Autodesk Inventor part; units mm, degrees
(part 5 of 13)
  line L1929 (20.935, 0.83) -> (20.6882, 0.83) construction
  spline S605 degree 3 poles (20.6882, 0.83) (20.4415, 0.83) (20.2414, 0.6299) (20.2414, 0.3832) knots 0 0 0 0 1 1 1 1
  line L1930 (20.6882, 0.83) -> (20.4415, 0.83) construction
  line L1931 (20.4415, 0.83) -> (20.2414, 0.6299) construction
  line L1932 (20.2414, 0.6299) -> (20.2414, 0.3832) construction
  spline S606 degree 3 poles (20.2414, 0.3832) (20.2414, 0.1364) (20.4415, -0.0639) (20.6882, -0.0639) knots 0 0 0 0 1 1 1 1
  line L1933 (20.2414, 0.3832) -> (20.2414, 0.1364) construction
  line L1934 (20.2414, 0.1364) -> (20.4415, -0.0639) construction
  line L1935 (20.4415, -0.0639) -> (20.6882, -0.0639) construction
  spline S607 degree 3 poles (20.6882, -0.0639) (20.935, -0.0639) (21.1353, 0.1364) (21.1353, 0.3832) knots 0 0 0 0 1 1 1 1
  line L1936 (20.6882, -0.0639) -> (20.935, -0.0639) construction
  line L1937 (20.935, -0.0639) -> (21.1353, 0.1364) construction
  line L1938 (21.1353, 0.1364) -> (21.1353, 0.3832) construction
  spline S608 degree 3 poles (19.8582, 5.4914) (19.8582, 5.7382) (19.658, 5.9382) (19.4112, 5.9382) knots 0 0 0 0 1 1 1 1
  line L1939 (19.8582, 5.4914) -> (19.8582, 5.7382) construction
  line L1940 (19.8582, 5.7382) -> (19.658, 5.9382) construction
  line L1941 (19.658, 5.9382) -> (19.4112, 5.9382) construction
  spline S609 degree 3 poles (19.4112, 5.9382) (19.1644, 5.9382) (18.9643, 5.7382) (18.9643, 5.4914) knots 0 0 0 0 1 1 1 1
  line L1942 (19.4112, 5.9382) -> (19.1644, 5.9382) construction
  line L1943 (19.1644, 5.9382) -> (18.9643, 5.7382) construction
  line L1944 (18.9643, 5.7382) -> (18.9643, 5.4914) construction
  spline S610 degree 3 poles (18.9643, 5.4914) (18.9643, 5.2446) (19.1644, 5.0443) (19.4112, 5.0443) knots 0 0 0 0 1 1 1 1
  line L1945 (18.9643, 5.4914) -> (18.9643, 5.2446) construction
  line L1946 (18.9643, 5.2446) -> (19.1644, 5.0443) construction
  line L1947 (19.1644, 5.0443) -> (19.4112, 5.0443) construction
  spline S611 degree 3 poles (19.4112, 5.0443) (19.658, 5.0443) (19.8582, 5.2446) (19.8582, 5.4914) knots 0 0 0 0 1 1 1 1
  line L1948 (19.4112, 5.0443) -> (19.658, 5.0443) construction
  line L1949 (19.658, 5.0443) -> (19.8582, 5.2446) construction
  line L1950 (19.8582, 5.2446) -> (19.8582, 5.4914) construction
  spline S612 degree 3 poles (19.8582, 8.0455) (19.8582, 8.2923) (19.658, 8.4923) (19.4112, 8.4923) knots 0 0 0 0 1 1 1 1
  line L1951 (19.8582, 8.0455) -> (19.8582, 8.2923) construction
  line L1952 (19.8582, 8.2923) -> (19.658, 8.4923) construction
  line L1953 (19.658, 8.4923) -> (19.4112, 8.4923) construction
  spline S613 degree 3 poles (19.4112, 8.4923) (19.1644, 8.4923) (18.9643, 8.2923) (18.9643, 8.0455) knots 0 0 0 0 1 1 1 1
  line L1954 (19.4112, 8.4923) -> (19.1644, 8.4923) construction
  line L1955 (19.1644, 8.4923) -> (18.9643, 8.2923) construction
  line L1956 (18.9643, 8.2923) -> (18.9643, 8.0455) construction
  spline S614 degree 3 poles (18.9643, 8.0455) (18.9643, 7.7987) (19.1644, 7.5984) (19.4112, 7.5984) knots 0 0 0 0 1 1 1 1
  line L1957 (18.9643, 8.0455) -> (18.9643, 7.7987) construction
  line L1958 (18.9643, 7.7987) -> (19.1644, 7.5984) construction
  line L1959 (19.1644, 7.5984) -> (19.4112, 7.5984) construction
  spline S615 degree 3 poles (19.4112, 7.5984) (19.658, 7.5984) (19.8582, 7.7987) (19.8582, 8.0455) knots 0 0 0 0 1 1 1 1
  line L1960 (19.4112, 7.5984) -> (19.658, 7.5984) construction
  line L1961 (19.658, 7.5984) -> (19.8582, 7.7987) construction
  line L1962 (19.8582, 7.7987) -> (19.8582, 8.0455) construction
  spline S616 degree 3 poles (19.8582, 10.5996) (19.8582, 10.8464) (19.658, 11.0465) (19.4112, 11.0465) knots 0 0 0 0 1 1 1 1
  line L1963 (19.8582, 10.5996) -> (19.8582, 10.8464) construction
  line L1964 (19.8582, 10.8464) -> (19.658, 11.0465) construction
  line L1965 (19.658, 11.0465) -> (19.4112, 11.0465) construction
  spline S617 degree 3 poles (19.4112, 11.0465) (19.1644, 11.0465) (18.9643, 10.8464) (18.9643, 10.5996) knots 0 0 0 0 1 1 1 1
  line L1966 (19.4112, 11.0465) -> (19.1644, 11.0465) construction
  line L1967 (19.1644, 11.0465) -> (18.9643, 10.8464) construction
  line L1968 (18.9643, 10.8464) -> (18.9643, 10.5996) construction
  spline S618 degree 3 poles (18.9643, 10.5996) (18.9643, 10.3528) (19.1644, 10.1525) (19.4112, 10.1525) knots 0 0 0 0 1 1 1 1
  line L1969 (18.9643, 10.5996) -> (18.9643, 10.3528) construction
  line L1970 (18.9643, 10.3528) -> (19.1644, 10.1525) construction
  line L1971 (19.1644, 10.1525) -> (19.4112, 10.1525) construction
  spline S619 degree 3 poles (19.4112, 10.1525) (19.658, 10.1525) (19.8582, 10.3528) (19.8582, 10.5996) knots 0 0 0 0 1 1 1 1
  line L1972 (19.4112, 10.1525) -> (19.658, 10.1525) construction
  line L1973 (19.658, 10.1525) -> (19.8582, 10.3528) construction
  line L1974 (19.8582, 10.3528) -> (19.8582, 10.5996) construction
  spline S620 degree 3 poles (22.7955, 11.7489) (22.7955, 11.9957) (22.5952, 12.1959) (22.3485, 12.1959) knots 0 0 0 0 1 1 1 1
  line L1975 (22.7955, 11.7489) -> (22.7955, 11.9957) construction
  line L1976 (22.7955, 11.9957) -> (22.5952, 12.1959) construction
  line L1977 (22.5952, 12.1959) -> (22.3485, 12.1959) construction
  spline S621 degree 3 poles (22.3485, 12.1959) (22.1017, 12.1959) (21.9014, 11.9957) (21.9014, 11.7489) knots 0 0 0 0 1 1 1 1
  line L1978 (22.3485, 12.1959) -> (22.1017, 12.1959) construction
  line L1979 (22.1017, 12.1959) -> (21.9014, 11.9957) construction
  line L1980 (21.9014, 11.9957) -> (21.9014, 11.7489) construction
  spline S622 degree 3 poles (21.9014, 11.7489) (21.9014, 11.5021) (22.1017, 11.302) (22.3485, 11.302) knots 0 0 0 0 1 1 1 1
  line L1981 (21.9014, 11.7489) -> (21.9014, 11.5021) construction
  line L1982 (21.9014, 11.5021) -> (22.1017, 11.302) construction
  line L1983 (22.1017, 11.302) -> (22.3485, 11.302) construction
  spline S623 degree 3 poles (22.3485, 11.302) (22.5952, 11.302) (22.7955, 11.5021) (22.7955, 11.7489) knots 0 0 0 0 1 1 1 1
  line L1984 (22.3485, 11.302) -> (22.5952, 11.302) construction
  line L1985 (22.5952, 11.302) -> (22.7955, 11.5021) construction
  line L1986 (22.7955, 11.5021) -> (22.7955, 11.7489) construction
  spline S624 degree 3 poles (25.3496, 11.7489) (25.3496, 11.9957) (25.1494, 12.1959) (24.9026, 12.1959) knots 0 0 0 0 1 1 1 1
  line L1987 (25.3496, 11.7489) -> (25.3496, 11.9957) construction
  line L1988 (25.3496, 11.9957) -> (25.1494, 12.1959) construction
  line L1989 (25.1494, 12.1959) -> (24.9026, 12.1959) construction
  spline S625 degree 3 poles (24.9026, 12.1959) (24.6558, 12.1959) (24.4555, 11.9957) (24.4555, 11.7489) knots 0 0 0 0 1 1 1 1
  line L1990 (24.9026, 12.1959) -> (24.6558, 12.1959) construction
  line L1991 (24.6558, 12.1959) -> (24.4555, 11.9957) construction
  line L1992 (24.4555, 11.9957) -> (24.4555, 11.7489) construction
  spline S626 degree 3 poles (24.4555, 11.7489) (24.4555, 11.5021) (24.6558, 11.302) (24.9026, 11.302) knots 0 0 0 0 1 1 1 1
  line L1993 (24.4555, 11.7489) -> (24.4555, 11.5021) construction
  line L1994 (24.4555, 11.5021) -> (24.6558, 11.302) construction
  line L1995 (24.6558, 11.302) -> (24.9026, 11.302) construction
  spline S627 degree 3 poles (24.9026, 11.302) (25.1494, 11.302) (25.3496, 11.5021) (25.3496, 11.7489) knots 0 0 0 0 1 1 1 1
  line L1996 (24.9026, 11.302) -> (25.1494, 11.302) construction
  line L1997 (25.1494, 11.302) -> (25.3496, 11.5021) construction
  line L1998 (25.3496, 11.5021) -> (25.3496, 11.7489) construction
  spline S628 degree 3 poles (22.7955, 14.303) (22.7955, 14.5498) (22.5952, 14.75) (22.3485, 14.75) knots 0 0 0 0 1 1 1 1
  line L1999 (22.7955, 14.303) -> (22.7955, 14.5498) construction
  line L2000 (22.7955, 14.5498) -> (22.5952, 14.75) construction
  line L2001 (22.5952, 14.75) -> (22.3485, 14.75) construction
  spline S629 degree 3 poles (22.3485, 14.75) (22.1017, 14.75) (21.9014, 14.5498) (21.9014, 14.303) knots 0 0 0 0 1 1 1 1
  line L2002 (22.3485, 14.75) -> (22.1017, 14.75) construction
  line L2003 (22.1017, 14.75) -> (21.9014, 14.5498) construction
  line L2004 (21.9014, 14.5498) -> (21.9014, 14.303) construction
  spline S630 degree 3 poles (21.9014, 14.303) (21.9014, 14.0562) (22.1017, 13.8561) (22.3485, 13.8561) knots 0 0 0 0 1 1 1 1
  line L2005 (21.9014, 14.303) -> (21.9014, 14.0562) construction
  line L2006 (21.9014, 14.0562) -> (22.1017, 13.8561) construction
  line L2007 (22.1017, 13.8561) -> (22.3485, 13.8561) construction
  spline S631 degree 3 poles (22.3485, 13.8561) (22.5952, 13.8561) (22.7955, 14.0562) (22.7955, 14.303) knots 0 0 0 0 1 1 1 1
  line L2008 (22.3485, 13.8561) -> (22.5952, 13.8561) construction
  line L2009 (22.5952, 13.8561) -> (22.7955, 14.0562) construction
  line L2010 (22.7955, 14.0562) -> (22.7955, 14.303) construction
  spline S632 degree 3 poles (25.3496, 14.303) (25.3496, 14.5498) (25.1494, 14.75) (24.9026, 14.75) knots 0 0 0 0 1 1 1 1
  line L2011 (25.3496, 14.303) -> (25.3496, 14.5498) construction
  line L2012 (25.3496, 14.5498) -> (25.1494, 14.75) construction
  line L2013 (25.1494, 14.75) -> (24.9026, 14.75) construction
  spline S633 degree 3 poles (24.9026, 14.75) (24.6558, 14.75) (24.4555, 14.5498) (24.4555, 14.303) knots 0 0 0 0 1 1 1 1
  line L2014 (24.9026, 14.75) -> (24.6558, 14.75) construction
  line L2015 (24.6558, 14.75) -> (24.4555, 14.5498) construction
  line L2016 (24.4555, 14.5498) -> (24.4555, 14.303) construction
  spline S634 degree 3 poles (24.4555, 14.303) (24.4555, 14.0562) (24.6558, 13.8561) (24.9026, 13.8561) knots 0 0 0 0 1 1 1 1
  line L2017 (24.4555, 14.303) -> (24.4555, 14.0562) construction
  line L2018 (24.4555, 14.0562) -> (24.6558, 13.8561) construction
  line L2019 (24.6558, 13.8561) -> (24.9026, 13.8561) construction
  spline S635 degree 3 poles (24.9026, 13.8561) (25.1494, 13.8561) (25.3496, 14.0562) (25.3496, 14.303) knots 0 0 0 0 1 1 1 1
  line L2020 (24.9026, 13.8561) -> (25.1494, 13.8561) construction
  line L2021 (25.1494, 13.8561) -> (25.3496, 14.0562) construction
  line L2022 (25.3496, 14.0562) -> (25.3496, 14.303) construction
  spline S636 degree 3 poles (17.3041, 5.4914) (17.3041, 5.7382) (17.1039, 5.9382) (16.8571, 5.9382) knots 0 0 0 0 1 1 1 1
  line L2023 (17.3041, 5.4914) -> (17.3041, 5.7382) construction
  line L2024 (17.3041, 5.7382) -> (17.1039, 5.9382) construction
  line L2025 (17.1039, 5.9382) -> (16.8571, 5.9382) construction
  spline S637 degree 3 poles (16.8571, 5.9382) (16.6103, 5.9382) (16.4102, 5.7382) (16.4102, 5.4914) knots 0 0 0 0 1 1 1 1
  line L2026 (16.8571, 5.9382) -> (16.6103, 5.9382) construction
  line L2027 (16.6103, 5.9382) -> (16.4102, 5.7382) construction
  line L2028 (16.4102, 5.7382) -> (16.4102, 5.4914) construction
  spline S638 degree 3 poles (16.4102, 5.4914) (16.4102, 5.2446) (16.6103, 5.0443) (16.8571, 5.0443) knots 0 0 0 0 1 1 1 1
  line L2029 (16.4102, 5.4914) -> (16.4102, 5.2446) construction
  line L2030 (16.4102, 5.2446) -> (16.6103, 5.0443) construction
  line L2031 (16.6103, 5.0443) -> (16.8571, 5.0443) construction
  spline S639 degree 3 poles (16.8571, 5.0443) (17.1039, 5.0443) (17.3041, 5.2446) (17.3041, 5.4914) knots 0 0 0 0 1 1 1 1
  line L2032 (16.8571, 5.0443) -> (17.1039, 5.0443) construction
  line L2033 (17.1039, 5.0443) -> (17.3041, 5.2446) construction
  line L2034 (17.3041, 5.2446) -> (17.3041, 5.4914) construction
  spline S640 degree 3 poles (14.75, 5.4914) (14.75, 5.7382) (14.5498, 5.9382) (14.303, 5.9382) knots 0 0 0 0 1 1 1 1
  line L2035 (14.75, 5.4914) -> (14.75, 5.7382) construction
  line L2036 (14.75, 5.7382) -> (14.5498, 5.9382) construction
  line L2037 (14.5498, 5.9382) -> (14.303, 5.9382) construction
  spline S641 degree 3 poles (14.303, 5.9382) (14.0562, 5.9382) (13.8561, 5.7382) (13.8561, 5.4914) knots 0 0 0 0 1 1 1 1
  line L2038 (14.303, 5.9382) -> (14.0562, 5.9382) construction
  line L2039 (14.0562, 5.9382) -> (13.8561, 5.7382) construction
  line L2040 (13.8561, 5.7382) -> (13.8561, 5.4914) construction
  spline S642 degree 3 poles (13.8561, 5.4914) (13.8561, 5.2446) (14.0562, 5.0443) (14.303, 5.0443) knots 0 0 0 0 1 1 1 1
  line L2041 (13.8561, 5.4914) -> (13.8561, 5.2446) construction
  line L2042 (13.8561, 5.2446) -> (14.0562, 5.0443) construction
  line L2043 (14.0562, 5.0443) -> (14.303, 5.0443) construction
  spline S643 degree 3 poles (14.303, 5.0443) (14.5498, 5.0443) (14.75, 5.2446) (14.75, 5.4914) knots 0 0 0 0 1 1 1 1
  line L2044 (14.303, 5.0443) -> (14.5498, 5.0443) construction
  line L2045 (14.5498, 5.0443) -> (14.75, 5.2446) construction
  line L2046 (14.75, 5.2446) -> (14.75, 5.4914) construction
  spline S644 degree 3 poles (17.3041, 8.0455) (17.3041, 8.2923) (17.1039, 8.4923) (16.8571, 8.4923) knots 0 0 0 0 1 1 1 1
  line L2047 (17.3041, 8.0455) -> (17.3041, 8.2923) construction
  line L2048 (17.3041, 8.2923) -> (17.1039, 8.4923) construction
  line L2049 (17.1039, 8.4923) -> (16.8571, 8.4923) construction
  spline S645 degree 3 poles (16.8571, 8.4923) (16.6103, 8.4923) (16.4102, 8.2923) (16.4102, 8.0455) knots 0 0 0 0 1 1 1 1
  line L2050 (16.8571, 8.4923) -> (16.6103, 8.4923) construction
  line L2051 (16.6103, 8.4923) -> (16.4102, 8.2923) construction
  line L2052 (16.4102, 8.2923) -> (16.4102, 8.0455) construction
  spline S646 degree 3 poles (16.4102, 8.0455) (16.4102, 7.7987) (16.6103, 7.5984) (16.8571, 7.5984) knots 0 0 0 0 1 1 1 1
  line L2053 (16.4102, 8.0455) -> (16.4102, 7.7987) construction
  line L2054 (16.4102, 7.7987) -> (16.6103, 7.5984) construction
  line L2055 (16.6103, 7.5984) -> (16.8571, 7.5984) construction
  spline S647 degree 3 poles (16.8571, 7.5984) (17.1039, 7.5984) (17.3041, 7.7987) (17.3041, 8.0455) knots 0 0 0 0 1 1 1 1
  line L2056 (16.8571, 7.5984) -> (17.1039, 7.5984) construction
  line L2057 (17.1039, 7.5984) -> (17.3041, 7.7987) construction
  line L2058 (17.3041, 7.7987) -> (17.3041, 8.0455) construction
  spline S648 degree 3 poles (17.3041, 10.5996) (17.3041, 10.8464) (17.1039, 11.0465) (16.8571, 11.0465) knots 0 0 0 0 1 1 1 1
  line L2059 (17.3041, 10.5996) -> (17.3041, 10.8464) construction
  line L2060 (17.3041, 10.8464) -> (17.1039, 11.0465) construction
  line L2061 (17.1039, 11.0465) -> (16.8571, 11.0465) construction
  spline S649 degree 3 poles (16.8571, 11.0465) (16.6103, 11.0465) (16.4102, 10.8464) (16.4102, 10.5996) knots 0 0 0 0 1 1 1 1
  line L2062 (16.8571, 11.0465) -> (16.6103, 11.0465) construction
  line L2063 (16.6103, 11.0465) -> (16.4102, 10.8464) construction
  line L2064 (16.4102, 10.8464) -> (16.4102, 10.5996) construction
  spline S650 degree 3 poles (16.4102, 10.5996) (16.4102, 10.3528) (16.6103, 10.1525) (16.8571, 10.1525) knots 0 0 0 0 1 1 1 1
  line L2065 (16.4102, 10.5996) -> (16.4102, 10.3528) construction
  line L2066 (16.4102, 10.3528) -> (16.6103, 10.1525) construction
  line L2067 (16.6103, 10.1525) -> (16.8571, 10.1525) construction
  spline S651 degree 3 poles (16.8571, 10.1525) (17.1039, 10.1525) (17.3041, 10.3528) (17.3041, 10.5996) knots 0 0 0 0 1 1 1 1
  line L2068 (16.8571, 10.1525) -> (17.1039, 10.1525) construction
  line L2069 (17.1039, 10.1525) -> (17.3041, 10.3528) construction
  line L2070 (17.3041, 10.3528) -> (17.3041, 10.5996) construction
  spline S652 degree 3 poles (17.3041, 13.1537) (17.3041, 13.4005) (17.1039, 13.6006) (16.8571, 13.6006) knots 0 0 0 0 1 1 1 1
  line L2071 (17.3041, 13.1537) -> (17.3041, 13.4005) construction
  line L2072 (17.3041, 13.4005) -> (17.1039, 13.6006) construction
  line L2073 (17.1039, 13.6006) -> (16.8571, 13.6006) construction
  spline S653 degree 3 poles (16.8571, 13.6006) (16.6103, 13.6006) (16.4102, 13.4005) (16.4102, 13.1537) knots 0 0 0 0 1 1 1 1
  line L2074 (16.8571, 13.6006) -> (16.6103, 13.6006) construction
  line L2075 (16.6103, 13.6006) -> (16.4102, 13.4005) construction
  line L2076 (16.4102, 13.4005) -> (16.4102, 13.1537) construction
  spline S654 degree 3 poles (16.4102, 13.1537) (16.4102, 12.9069) (16.6103, 12.7067) (16.8571, 12.7067) knots 0 0 0 0 1 1 1 1
  line L2077 (16.4102, 13.1537) -> (16.4102, 12.9069) construction
  line L2078 (16.4102, 12.9069) -> (16.6103, 12.7067) construction
  line L2079 (16.6103, 12.7067) -> (16.8571, 12.7067) construction
  spline S655 degree 3 poles (16.8571, 12.7067) (17.1039, 12.7067) (17.3041, 12.9069) (17.3041, 13.1537) knots 0 0 0 0 1 1 1 1
  line L2080 (16.8571, 12.7067) -> (17.1039, 12.7067) construction
  line L2081 (17.1039, 12.7067) -> (17.3041, 12.9069) construction
  line L2082 (17.3041, 12.9069) -> (17.3041, 13.1537) construction
  spline S656 degree 3 poles (17.3041, 15.7078) (17.3041, 15.9546) (17.1039, 16.1547) (16.8571, 16.1547) knots 0 0 0 0 1 1 1 1
  line L2083 (17.3041, 15.7078) -> (17.3041, 15.9546) construction
  line L2084 (17.3041, 15.9546) -> (17.1039, 16.1547) construction
  line L2085 (17.1039, 16.1547) -> (16.8571, 16.1547) construction
  spline S657 degree 3 poles (16.8571, 16.1547) (16.6103, 16.1547) (16.4102, 15.9546) (16.4102, 15.7078) knots 0 0 0 0 1 1 1 1
  line L2086 (16.8571, 16.1547) -> (16.6103, 16.1547) construction
  line L2087 (16.6103, 16.1547) -> (16.4102, 15.9546) construction
  line L2088 (16.4102, 15.9546) -> (16.4102, 15.7078) construction
  spline S658 degree 3 poles (16.4102, 15.7078) (16.4102, 15.461) (16.6103, 15.2608) (16.8571, 15.2608) knots 0 0 0 0 1 1 1 1
  line L2089 (16.4102, 15.7078) -> (16.4102, 15.461) construction
  line L2090 (16.4102, 15.461) -> (16.6103, 15.2608) construction
  line L2091 (16.6103, 15.2608) -> (16.8571, 15.2608) construction
  spline S659 degree 3 poles (16.8571, 15.2608) (17.1039, 15.2608) (17.3041, 15.461) (17.3041, 15.7078) knots 0 0 0 0 1 1 1 1
  line L2092 (16.8571, 15.2608) -> (17.1039, 15.2608) construction
  line L2093 (17.1039, 15.2608) -> (17.3041, 15.461) construction
  line L2094 (17.3041, 15.461) -> (17.3041, 15.7078) construction
  spline S660 degree 3 poles (17.3041, 18.2619) (17.3041, 18.5087) (17.1039, 18.7088) (16.8571, 18.7088) knots 0 0 0 0 1 1 1 1
  line L2095 (17.3041, 18.2619) -> (17.3041, 18.5087) construction
  line L2096 (17.3041, 18.5087) -> (17.1039, 18.7088) construction
  line L2097 (17.1039, 18.7088) -> (16.8571, 18.7088) construction
  spline S661 degree 3 poles (16.8571, 18.7088) (16.6103, 18.7088) (16.4102, 18.5087) (16.4102, 18.2619) knots 0 0 0 0 1 1 1 1
  line L2098 (16.8571, 18.7088) -> (16.6103, 18.7088) construction
  line L2099 (16.6103, 18.7088) -> (16.4102, 18.5087) construction
  line L2100 (16.4102, 18.5087) -> (16.4102, 18.2619) construction
  spline S662 degree 3 poles (16.4102, 18.2619) (16.4102, 18.0151) (16.6103, 17.8149) (16.8571, 17.8149) knots 0 0 0 0 1 1 1 1
  line L2101 (16.4102, 18.2619) -> (16.4102, 18.0151) construction
  line L2102 (16.4102, 18.0151) -> (16.6103, 17.8149) construction
  line L2103 (16.6103, 17.8149) -> (16.8571, 17.8149) construction
  spline S663 degree 3 poles (16.8571, 17.8149) (17.1039, 17.8149) (17.3041, 18.0151) (17.3041, 18.2619) knots 0 0 0 0 1 1 1 1
  line L2104 (16.8571, 17.8149) -> (17.1039, 17.8149) construction
  line L2105 (17.1039, 17.8149) -> (17.3041, 18.0151) construction
  line L2106 (17.3041, 18.0151) -> (17.3041, 18.2619) construction
  spline S664 degree 3 poles (17.3041, 20.816) (17.3041, 21.0628) (17.1039, 21.2629) (16.8571, 21.2629) knots 0 0 0 0 1 1 1 1
  line L2107 (17.3041, 20.816) -> (17.3041, 21.0628) construction
  line L2108 (17.3041, 21.0628) -> (17.1039, 21.2629) construction
  line L2109 (17.1039, 21.2629) -> (16.8571, 21.2629) construction
  spline S665 degree 3 poles (16.8571, 21.2629) (16.6103, 21.2629) (16.4102, 21.0628) (16.4102, 20.816) knots 0 0 0 0 1 1 1 1
  line L2110 (16.8571, 21.2629) -> (16.6103, 21.2629) construction
  line L2111 (16.6103, 21.2629) -> (16.4102, 21.0628) construction
  line L2112 (16.4102, 21.0628) -> (16.4102, 20.816) construction
  spline S666 degree 3 poles (16.4102, 20.816) (16.4102, 20.5692) (16.6103, 20.369) (16.8571, 20.369) knots 0 0 0 0 1 1 1 1
  line L2113 (16.4102, 20.816) -> (16.4102, 20.5692) construction
  line L2114 (16.4102, 20.5692) -> (16.6103, 20.369) construction
  line L2115 (16.6103, 20.369) -> (16.8571, 20.369) construction
  spline S667 degree 3 poles (16.8571, 20.369) (17.1039, 20.369) (17.3041, 20.5692) (17.3041, 20.816) knots 0 0 0 0 1 1 1 1
  line L2116 (16.8571, 20.369) -> (17.1039, 20.369) construction
  line L2117 (17.1039, 20.369) -> (17.3041, 20.5692) construction
  line L2118 (17.3041, 20.5692) -> (17.3041, 20.816) construction
  spline S668 degree 3 poles (19.8582, 13.1537) (19.8582, 13.4005) (19.658, 13.6006) (19.4112, 13.6006) knots 0 0 0 0 1 1 1 1
  line L2119 (19.8582, 13.1537) -> (19.8582, 13.4005) construction
  line L2120 (19.8582, 13.4005) -> (19.658, 13.6006) construction
  line L2121 (19.658, 13.6006) -> (19.4112, 13.6006) construction
  spline S669 degree 3 poles (19.4112, 13.6006) (19.1644, 13.6006) (18.9643, 13.4005) (18.9643, 13.1537) knots 0 0 0 0 1 1 1 1
  line L2122 (19.4112, 13.6006) -> (19.1644, 13.6006) construction
  line L2123 (19.1644, 13.6006) -> (18.9643, 13.4005) construction
  line L2124 (18.9643, 13.4005) -> (18.9643, 13.1537) construction
  spline S670 degree 3 poles (18.9643, 13.1537) (18.9643, 12.9069) (19.1644, 12.7067) (19.4112, 12.7067) knots 0 0 0 0 1 1 1 1
  line L2125 (18.9643, 13.1537) -> (18.9643, 12.9069) construction
  line L2126 (18.9643, 12.9069) -> (19.1644, 12.7067) construction
  line L2127 (19.1644, 12.7067) -> (19.4112, 12.7067) construction
  spline S671 degree 3 poles (19.4112, 12.7067) (19.658, 12.7067) (19.8582, 12.9069) (19.8582, 13.1537) knots 0 0 0 0 1 1 1 1
  line L2128 (19.4112, 12.7067) -> (19.658, 12.7067) construction
  line L2129 (19.658, 12.7067) -> (19.8582, 12.9069) construction
  line L2130 (19.8582, 12.9069) -> (19.8582, 13.1537) construction
  spline S672 degree 3 poles (19.8582, 15.7078) (19.8582, 15.9546) (19.658, 16.1547) (19.4112, 16.1547) knots 0 0 0 0 1 1 1 1
  line L2131 (19.8582, 15.7078) -> (19.8582, 15.9546) construction
  line L2132 (19.8582, 15.9546) -> (19.658, 16.1547) construction
  line L2133 (19.658, 16.1547) -> (19.4112, 16.1547) construction
  spline S673 degree 3 poles (19.4112, 16.1547) (19.1644, 16.1547) (18.9643, 15.9546) (18.9643, 15.7078) knots 0 0 0 0 1 1 1 1
  line L2134 (19.4112, 16.1547) -> (19.1644, 16.1547) construction
  line L2135 (19.1644, 16.1547) -> (18.9643, 15.9546) construction
  line L2136 (18.9643, 15.9546) -> (18.9643, 15.7078) construction
  spline S674 degree 3 poles (18.9643, 15.7078) (18.9643, 15.461) (19.1644, 15.2608) (19.4112, 15.2608) knots 0 0 0 0 1 1 1 1
  line L2137 (18.9643, 15.7078) -> (18.9643, 15.461) construction
  line L2138 (18.9643, 15.461) -> (19.1644, 15.2608) construction
  line L2139 (19.1644, 15.2608) -> (19.4112, 15.2608) construction
  spline S675 degree 3 poles (19.4112, 15.2608) (19.658, 15.2608) (19.8582, 15.461) (19.8582, 15.7078) knots 0 0 0 0 1 1 1 1
  line L2140 (19.4112, 15.2608) -> (19.658, 15.2608) construction
  line L2141 (19.658, 15.2608) -> (19.8582, 15.461) construction
  line L2142 (19.8582, 15.461) -> (19.8582, 15.7078) construction
  spline S676 degree 3 poles (19.8582, 18.2619) (19.8582, 18.5087) (19.658, 18.7088) (19.4112, 18.7088) knots 0 0 0 0 1 1 1 1
  line L2143 (19.8582, 18.2619) -> (19.8582, 18.5087) construction
  line L2144 (19.8582, 18.5087) -> (19.658, 18.7088) construction
  line L2145 (19.658, 18.7088) -> (19.4112, 18.7088) construction
  spline S677 degree 3 poles (19.4112, 18.7088) (19.1644, 18.7088) (18.9643, 18.5087) (18.9643, 18.2619) knots 0 0 0 0 1 1 1 1
  line L2146 (19.4112, 18.7088) -> (19.1644, 18.7088) construction
  line L2147 (19.1644, 18.7088) -> (18.9643, 18.5087) construction
  line L2148 (18.9643, 18.5087) -> (18.9643, 18.2619) construction
  spline S678 degree 3 poles (18.9643, 18.2619) (18.9643, 18.0151) (19.1644, 17.8149) (19.4112, 17.8149) knots 0 0 0 0 1 1 1 1
  line L2149 (18.9643, 18.2619) -> (18.9643, 18.0151) construction
  line L2150 (18.9643, 18.0151) -> (19.1644, 17.8149) construction
  line L2151 (19.1644, 17.8149) -> (19.4112, 17.8149) construction
  spline S679 degree 3 poles (19.4112, 17.8149) (19.658, 17.8149) (19.8582, 18.0151) (19.8582, 18.2619) knots 0 0 0 0 1 1 1 1
  line L2152 (19.4112, 17.8149) -> (19.658, 17.8149) construction
  line L2153 (19.658, 17.8149) -> (19.8582, 18.0151) construction
  line L2154 (19.8582, 18.0151) -> (19.8582, 18.2619) construction
  spline S680 degree 3 poles (19.8582, 20.816) (19.8582, 21.0628) (19.658, 21.2629) (19.4112, 21.2629) knots 0 0 0 0 1 1 1 1
  line L2155 (19.8582, 20.816) -> (19.8582, 21.0628) construction
  line L2156 (19.8582, 21.0628) -> (19.658, 21.2629) construction
  line L2157 (19.658, 21.2629) -> (19.4112, 21.2629) construction
  spline S681 degree 3 poles (19.4112, 21.2629) (19.1644, 21.2629) (18.9643, 21.0628) (18.9643, 20.816) knots 0 0 0 0 1 1 1 1
  line L2158 (19.4112, 21.2629) -> (19.1644, 21.2629) construction
  line L2159 (19.1644, 21.2629) -> (18.9643, 21.0628) construction
  line L2160 (18.9643, 21.0628) -> (18.9643, 20.816) construction
  spline S682 degree 3 poles (18.9643, 20.816) (18.9643, 20.5692) (19.1644, 20.369) (19.4112, 20.369) knots 0 0 0 0 1 1 1 1
  line L2161 (18.9643, 20.816) -> (18.9643, 20.5692) construction
  line L2162 (18.9643, 20.5692) -> (19.1644, 20.369) construction
  line L2163 (19.1644, 20.369) -> (19.4112, 20.369) construction
  spline S683 degree 3 poles (19.4112, 20.369) (19.658, 20.369) (19.8582, 20.5692) (19.8582, 20.816) knots 0 0 0 0 1 1 1 1
  line L2164 (19.4112, 20.369) -> (19.658, 20.369) construction
  line L2165 (19.658, 20.369) -> (19.8582, 20.5692) construction
  line L2166 (19.8582, 20.5692) -> (19.8582, 20.816) construction
  line L2167 (23.6255, 14.4308) -> (23.6255, 14.1754)
  line L2168 (4.0865, 34.8636) -> (50.0605, 34.8636)
  line L2169 (0.2554, 31.0325) -> (0.2554, 2.9373)
  line L2170 (53.8917, 31.0325) -> (53.8917, 2.9373)
  spline S684 degree 3 poles (50.0605, 34.8636) (52.1762, 34.8636) (53.8917, 33.1483) (53.8917, 31.0325) knots 0 0 0 0 1 1 1 1
  line L2171 (50.0605, 34.8636) -> (52.1762, 34.8636) construction
  line L2172 (52.1762, 34.8636) -> (53.8917, 33.1483) construction
  line L2173 (53.8917, 33.1483) -> (53.8917, 31.0325) construction
  spline S685 degree 3 poles (53.8917, 2.9373) (53.8917, 0.8214) (52.1762, -0.8939) (50.0605, -0.8939) knots 0 0 0 0 1 1 1 1
  line L2174 (53.8917, 2.9373) -> (53.8917, 0.8214) construction
  line L2175 (53.8917, 0.8214) -> (52.1762, -0.8939) construction
  line L2176 (52.1762, -0.8939) -> (50.0605, -0.8939) construction
  spline S686 degree 3 poles (4.0865, -0.8939) (1.9707, -0.8939) (0.2554, 0.8214) (0.2554, 2.9373) knots 0 0 0 0 1 1 1 1
  line L2177 (4.0865, -0.8939) -> (1.9707, -0.8939) construction
  line L2178 (1.9707, -0.8939) -> (0.2554, 0.8214) construction
  line L2179 (0.2554, 0.8214) -> (0.2554, 2.9373) construction
  spline S687 degree 3 poles (0.2554, 31.0325) (0.2554, 33.1483) (1.9707, 34.8636) (4.0865, 34.8636) knots 0 0 0 0 1 1 1 1
  line L2180 (0.2554, 31.0325) -> (0.2554, 33.1483) construction
  line L2181 (0.2554, 33.1483) -> (1.9707, 34.8636) construction
  line L2182 (1.9707, 34.8636) -> (4.0865, 34.8636) construction
  line L2183 (4.0865, -0.8939) -> (50.0605, -0.8939)
  spline S688 degree 3 poles (10.1653, 33.5866) (10.1653, 34.1226) (9.7308, 34.5571) (9.1948, 34.5571) knots 0 0 0 0 1 1 1 1
  line L2184 (10.1653, 33.5866) -> (10.1653, 34.1226) construction
  line L2185 (10.1653, 34.1226) -> (9.7308, 34.5571) construction
  line L2186 (9.7308, 34.5571) -> (9.1948, 34.5571) construction
  spline S689 degree 3 poles (9.1948, 34.5571) (8.6588, 34.5571) (8.2242, 34.1226) (8.2242, 33.5866) knots 0 0 0 0 1 1 1 1
  line L2187 (9.1948, 34.5571) -> (8.6588, 34.5571) construction
  line L2188 (8.6588, 34.5571) -> (8.2242, 34.1226) construction
  line L2189 (8.2242, 34.1226) -> (8.2242, 33.5866) construction
  spline S690 degree 3 poles (8.2242, 33.5866) (8.2242, 33.0506) (8.6588, 32.616) (9.1948, 32.616) knots 0 0 0 0 1 1 1 1
  line L2190 (8.2242, 33.5866) -> (8.2242, 33.0506) construction
  line L2191 (8.2242, 33.0506) -> (8.6588, 32.616) construction
  line L2192 (8.6588, 32.616) -> (9.1948, 32.616) construction
  spline S691 degree 3 poles (9.1948, 32.616) (9.7308, 32.616) (10.1653, 33.0506) (10.1653, 33.5866) knots 0 0 0 0 1 1 1 1
  line L2193 (9.1948, 32.616) -> (9.7308, 32.616) construction
  line L2194 (9.7308, 32.616) -> (10.1653, 33.0506) construction
  line L2195 (10.1653, 33.0506) -> (10.1653, 33.5866) construction
  spline S692 degree 3 poles (12.7194, 33.5866) (12.7194, 34.1226) (12.2849, 34.5571) (11.7489, 34.5571) knots 0 0 0 0 1 1 1 1
  line L2196 (12.7194, 33.5866) -> (12.7194, 34.1226) construction
  line L2197 (12.7194, 34.1226) -> (12.2849, 34.5571) construction
  line L2198 (12.2849, 34.5571) -> (11.7489, 34.5571) construction
  spline S693 degree 3 poles (11.7489, 34.5571) (11.2129, 34.5571) (10.7783, 34.1226) (10.7783, 33.5866) knots 0 0 0 0 1 1 1 1
  line L2199 (11.7489, 34.5571) -> (11.2129, 34.5571) construction
  line L2200 (11.2129, 34.5571) -> (10.7783, 34.1226) construction
  line L2201 (10.7783, 34.1226) -> (10.7783, 33.5866) construction
  spline S694 degree 3 poles (10.7783, 33.5866) (10.7783, 33.0506) (11.2129, 32.616) (11.7489, 32.616) knots 0 0 0 0 1 1 1 1
  line L2202 (10.7783, 33.5866) -> (10.7783, 33.0506) construction
  line L2203 (10.7783, 33.0506) -> (11.2129, 32.616) construction
  line L2204 (11.2129, 32.616) -> (11.7489, 32.616) construction
  spline S695 degree 3 poles (11.7489, 32.616) (12.2849, 32.616) (12.7194, 33.0506) (12.7194, 33.5866) knots 0 0 0 0 1 1 1 1
  line L2205 (11.7489, 32.616) -> (12.2849, 32.616) construction
  line L2206 (12.2849, 32.616) -> (12.7194, 33.0506) construction
  line L2207 (12.7194, 33.0506) -> (12.7194, 33.5866) construction
  spline S696 degree 3 poles (15.2735, 33.5866) (15.2735, 34.1226) (14.839, 34.5571) (14.303, 34.5571) knots 0 0 0 0 1 1 1 1
  line L2208 (15.2735, 33.5866) -> (15.2735, 34.1226) construction
  line L2209 (15.2735, 34.1226) -> (14.839, 34.5571) construction
  line L2210 (14.839, 34.5571) -> (14.303, 34.5571) construction
  spline S697 degree 3 poles (14.303, 34.5571) (13.767, 34.5571) (13.3324, 34.1226) (13.3324, 33.5866) knots 0 0 0 0 1 1 1 1
  line L2211 (14.303, 34.5571) -> (13.767, 34.5571) construction
  line L2212 (13.767, 34.5571) -> (13.3324, 34.1226) construction
  line L2213 (13.3324, 34.1226) -> (13.3324, 33.5866) construction
  spline S698 degree 3 poles (13.3324, 33.5866) (13.3324, 33.0506) (13.767, 32.616) (14.303, 32.616) knots 0 0 0 0 1 1 1 1
  line L2214 (13.3324, 33.5866) -> (13.3324, 33.0506) construction
  line L2215 (13.3324, 33.0506) -> (13.767, 32.616) construction
  line L2216 (13.767, 32.616) -> (14.303, 32.616) construction
  spline S699 degree 3 poles (14.303, 32.616) (14.839, 32.616) (15.2735, 33.0506) (15.2735, 33.5866) knots 0 0 0 0 1 1 1 1
  line L2217 (14.303, 32.616) -> (14.839, 32.616) construction
  line L2218 (14.839, 32.616) -> (15.2735, 33.0506) construction
  line L2219 (15.2735, 33.0506) -> (15.2735, 33.5866) construction
  spline S700 degree 3 poles (17.8276, 23.3701) (17.8276, 23.9061) (17.3931, 24.3407) (16.8571, 24.3407) knots 0 0 0 0 1 1 1 1
  line L2220 (17.8276, 23.3701) -> (17.8276, 23.9061) construction
  line L2221 (17.8276, 23.9061) -> (17.3931, 24.3407) construction
  line L2222 (17.3931, 24.3407) -> (16.8571, 24.3407) construction
  spline S701 degree 3 poles (16.8571, 24.3407) (16.3211, 24.3407) (15.8866, 23.9061) (15.8866, 23.3701) knots 0 0 0 0 1 1 1 1
  line L2223 (16.8571, 24.3407) -> (16.3211, 24.3407) construction
  line L2224 (16.3211, 24.3407) -> (15.8866, 23.9061) construction
  line L2225 (15.8866, 23.9061) -> (15.8866, 23.3701) construction
  spline S702 degree 3 poles (15.8866, 23.3701) (15.8866, 22.8341) (16.3211, 22.3996) (16.8571, 22.3996) knots 0 0 0 0 1 1 1 1
  line L2226 (15.8866, 23.3701) -> (15.8866, 22.8341) construction
  line L2227 (15.8866, 22.8341) -> (16.3211, 22.3996) construction
  line L2228 (16.3211, 22.3996) -> (16.8571, 22.3996) construction
  spline S703 degree 3 poles (16.8571, 22.3996) (17.3931, 22.3996) (17.8276, 22.8341) (17.8276, 23.3701) knots 0 0 0 0 1 1 1 1
  line L2229 (16.8571, 22.3996) -> (17.3931, 22.3996) construction
  line L2230 (17.3931, 22.3996) -> (17.8276, 22.8341) construction
  line L2231 (17.8276, 22.8341) -> (17.8276, 23.3701) construction
  spline S704 degree 3 poles (23.319, 22.2718) (23.319, 22.8078) (22.8844, 23.2424) (22.3485, 23.2424) knots 0 0 0 0 1 1 1 1
  line L2232 (23.319, 22.2718) -> (23.319, 22.8078) construction
  line L2233 (23.319, 22.8078) -> (22.8844, 23.2424) construction
  line L2234 (22.8844, 23.2424) -> (22.3485, 23.2424) construction
  spline S705 degree 3 poles (22.3485, 23.2424) (21.8125, 23.2424) (21.3779, 22.8078) (21.3779, 22.2718) knots 0 0 0 0 1 1 1 1
  line L2235 (22.3485, 23.2424) -> (21.8125, 23.2424) construction
  line L2236 (21.8125, 23.2424) -> (21.3779, 22.8078) construction
  line L2237 (21.3779, 22.8078) -> (21.3779, 22.2718) construction
  spline S706 degree 3 poles (21.3779, 22.2718) (21.3779, 21.7358) (21.8125, 21.3013) (22.3485, 21.3013) knots 0 0 0 0 1 1 1 1
  line L2238 (21.3779, 22.2718) -> (21.3779, 21.7358) construction
  line L2239 (21.3779, 21.7358) -> (21.8125, 21.3013) construction
  line L2240 (21.8125, 21.3013) -> (22.3485, 21.3013) construction
  spline S707 degree 3 poles (22.3485, 21.3013) (22.8844, 21.3013) (23.319, 21.7358) (23.319, 22.2718) knots 0 0 0 0 1 1 1 1
  line L2241 (22.3485, 21.3013) -> (22.8844, 21.3013) construction
  line L2242 (22.8844, 21.3013) -> (23.319, 21.7358) construction
  line L2243 (23.319, 21.7358) -> (23.319, 22.2718) construction
  spline S708 degree 3 poles (25.8731, 22.2718) (25.8731, 22.8078) (25.4385, 23.2424) (24.9026, 23.2424) knots 0 0 0 0 1 1 1 1
  line L2244 (25.8731, 22.2718) -> (25.8731, 22.8078) construction
  line L2245 (25.8731, 22.8078) -> (25.4385, 23.2424) construction
  line L2246 (25.4385, 23.2424) -> (24.9026, 23.2424) construction
  spline S709 degree 3 poles (24.9026, 23.2424) (24.3666, 23.2424) (23.932, 22.8078) (23.932, 22.2718) knots 0 0 0 0 1 1 1 1
  line L2247 (24.9026, 23.2424) -> (24.3666, 23.2424) construction
  line L2248 (24.3666, 23.2424) -> (23.932, 22.8078) construction
  line L2249 (23.932, 22.8078) -> (23.932, 22.2718) construction
  spline S710 degree 3 poles (23.932, 22.2718) (23.932, 21.7358) (24.3666, 21.3013) (24.9026, 21.3013) knots 0 0 0 0 1 1 1 1
  line L2250 (23.932, 22.2718) -> (23.932, 21.7358) construction
  line L2251 (23.932, 21.7358) -> (24.3666, 21.3013) construction
  line L2252 (24.3666, 21.3013) -> (24.9026, 21.3013) construction
  spline S711 degree 3 poles (24.9026, 21.3013) (25.4385, 21.3013) (25.8731, 21.7358) (25.8731, 22.2718) knots 0 0 0 0 1 1 1 1
  line L2253 (24.9026, 21.3013) -> (25.4385, 21.3013) construction
  line L2254 (25.4385, 21.3013) -> (25.8731, 21.7358) construction
  line L2255 (25.8731, 21.7358) -> (25.8731, 22.2718) construction
  spline S712 degree 3 poles (23.319, 24.8259) (23.319, 25.3619) (22.8844, 25.7965) (22.3485, 25.7965) knots 0 0 0 0 1 1 1 1
  line L2256 (23.319, 24.8259) -> (23.319, 25.3619) construction
  line L2257 (23.319, 25.3619) -> (22.8844, 25.7965) construction
  line L2258 (22.8844, 25.7965) -> (22.3485, 25.7965) construction
  spline S713 degree 3 poles (22.3485, 25.7965) (21.8125, 25.7965) (21.3779, 25.3619) (21.3779, 24.8259) knots 0 0 0 0 1 1 1 1
  line L2259 (22.3485, 25.7965) -> (21.8125, 25.7965) construction
  line L2260 (21.8125, 25.7965) -> (21.3779, 25.3619) construction
  line L2261 (21.3779, 25.3619) -> (21.3779, 24.8259) construction
  spline S714 degree 3 poles (21.3779, 24.8259) (21.3779, 24.2899) (21.8125, 23.8554) (22.3485, 23.8554) knots 0 0 0 0 1 1 1 1
  line L2262 (21.3779, 24.8259) -> (21.3779, 24.2899) construction
  line L2263 (21.3779, 24.2899) -> (21.8125, 23.8554) construction
  line L2264 (21.8125, 23.8554) -> (22.3485, 23.8554) construction
  spline S715 degree 3 poles (22.3485, 23.8554) (22.8844, 23.8554) (23.319, 24.2899) (23.319, 24.8259) knots 0 0 0 0 1 1 1 1
  line L2265 (22.3485, 23.8554) -> (22.8844, 23.8554) construction
  line L2266 (22.8844, 23.8554) -> (23.319, 24.2899) construction
  line L2267 (23.319, 24.2899) -> (23.319, 24.8259) construction
  spline S716 degree 3 poles (25.8731, 24.8259) (25.8731, 25.3619) (25.4385, 25.7965) (24.9026, 25.7965) knots 0 0 0 0 1 1 1 1
  line L2268 (25.8731, 24.8259) -> (25.8731, 25.3619) construction
  line L2269 (25.8731, 25.3619) -> (25.4385, 25.7965) construction
  line L2270 (25.4385, 25.7965) -> (24.9026, 25.7965) construction
  spline S717 degree 3 poles (24.9026, 25.7965) (24.3666, 25.7965) (23.932, 25.3619) (23.932, 24.8259) knots 0 0 0 0 1 1 1 1
  line L2271 (24.9026, 25.7965) -> (24.3666, 25.7965) construction
  line L2272 (24.3666, 25.7965) -> (23.932, 25.3619) construction
  line L2273 (23.932, 25.3619) -> (23.932, 24.8259) construction
  spline S718 degree 3 poles (23.932, 24.8259) (23.932, 24.2899) (24.3666, 23.8554) (24.9026, 23.8554) knots 0 0 0 0 1 1 1 1
  line L2274 (23.932, 24.8259) -> (23.932, 24.2899) construction
  line L2275 (23.932, 24.2899) -> (24.3666, 23.8554) construction
  line L2276 (24.3666, 23.8554) -> (24.9026, 23.8554) construction
  spline S719 degree 3 poles (24.9026, 23.8554) (25.4385, 23.8554) (25.8731, 24.2899) (25.8731, 24.8259) knots 0 0 0 0 1 1 1 1
  line L2277 (24.9026, 23.8554) -> (25.4385, 23.8554) construction
  line L2278 (25.4385, 23.8554) -> (25.8731, 24.2899) construction
  line L2279 (25.8731, 24.2899) -> (25.8731, 24.8259) construction
  spline S720 degree 3 poles (20.3818, 23.3701) (20.3818, 23.9061) (19.9472, 24.3407) (19.4112, 24.3407) knots 0 0 0 0 1 1 1 1
  line L2280 (20.3818, 23.3701) -> (20.3818, 23.9061) construction
  line L2281 (20.3818, 23.9061) -> (19.9472, 24.3407) construction
  line L2282 (19.9472, 24.3407) -> (19.4112, 24.3407) construction
  spline S721 degree 3 poles (19.4112, 24.3407) (18.8752, 24.3407) (18.4407, 23.9061) (18.4407, 23.3701) knots 0 0 0 0 1 1 1 1
  line L2283 (19.4112, 24.3407) -> (18.8752, 24.3407) construction
  line L2284 (18.8752, 24.3407) -> (18.4407, 23.9061) construction
  line L2285 (18.4407, 23.9061) -> (18.4407, 23.3701) construction
  spline S722 degree 3 poles (18.4407, 23.3701) (18.4407, 22.8341) (18.8752, 22.3996) (19.4112, 22.3996) knots 0 0 0 0 1 1 1 1
  line L2286 (18.4407, 23.3701) -> (18.4407, 22.8341) construction
  line L2287 (18.4407, 22.8341) -> (18.8752, 22.3996) construction
  line L2288 (18.8752, 22.3996) -> (19.4112, 22.3996) construction
  spline S723 degree 3 poles (19.4112, 22.3996) (19.9472, 22.3996) (20.3818, 22.8341) (20.3818, 23.3701) knots 0 0 0 0 1 1 1 1
  line L2289 (19.4112, 22.3996) -> (19.9472, 22.3996) construction
  line L2290 (19.9472, 22.3996) -> (20.3818, 22.8341) construction
  line L2291 (20.3818, 22.8341) -> (20.3818, 23.3701) construction
  spline S724 degree 3 poles (20.3818, 25.9242) (20.3818, 26.4602) (19.9472, 26.8948) (19.4112, 26.8948) knots 0 0 0 0 1 1 1 1
  line L2292 (20.3818, 25.9242) -> (20.3818, 26.4602) construction
  line L2293 (20.3818, 26.4602) -> (19.9472, 26.8948) construction
  line L2294 (19.9472, 26.8948) -> (19.4112, 26.8948) construction
  spline S725 degree 3 poles (19.4112, 26.8948) (18.8752, 26.8948) (18.4407, 26.4602) (18.4407, 25.9242) knots 0 0 0 0 1 1 1 1
  line L2295 (19.4112, 26.8948) -> (18.8752, 26.8948) construction
  line L2296 (18.8752, 26.8948) -> (18.4407, 26.4602) construction
  line L2297 (18.4407, 26.4602) -> (18.4407, 25.9242) construction
  spline S726 degree 3 poles (18.4407, 25.9242) (18.4407, 25.3882) (18.8752, 24.9537) (19.4112, 24.9537) knots 0 0 0 0 1 1 1 1
  line L2298 (18.4407, 25.9242) -> (18.4407, 25.3882) construction
  line L2299 (18.4407, 25.3882) -> (18.8752, 24.9537) construction
  line L2300 (18.8752, 24.9537) -> (19.4112, 24.9537) construction
  spline S727 degree 3 poles (19.4112, 24.9537) (19.9472, 24.9537) (20.3818, 25.3882) (20.3818, 25.9242) knots 0 0 0 0 1 1 1 1
  line L2301 (19.4112, 24.9537) -> (19.9472, 24.9537) construction
  line L2302 (19.9472, 24.9537) -> (20.3818, 25.3882) construction
  line L2303 (20.3818, 25.3882) -> (20.3818, 25.9242) construction
  spline S728 degree 3 poles (20.3818, 28.4784) (20.3818, 29.0143) (19.9472, 29.4489) (19.4112, 29.4489) knots 0 0 0 0 1 1 1 1
  line L2304 (20.3818, 28.4784) -> (20.3818, 29.0143) construction
  line L2305 (20.3818, 29.0143) -> (19.9472, 29.4489) construction
  line L2306 (19.9472, 29.4489) -> (19.4112, 29.4489) construction
  spline S729 degree 3 poles (19.4112, 29.4489) (18.8752, 29.4489) (18.4407, 29.0143) (18.4407, 28.4784) knots 0 0 0 0 1 1 1 1
  line L2307 (19.4112, 29.4489) -> (18.8752, 29.4489) construction
  line L2308 (18.8752, 29.4489) -> (18.4407, 29.0143) construction
  line L2309 (18.4407, 29.0143) -> (18.4407, 28.4784) construction
  spline S730 degree 3 poles (18.4407, 28.4784) (18.4407, 27.9423) (18.8752, 27.5078) (19.4112, 27.5078) knots 0 0 0 0 1 1 1 1
  line L2310 (18.4407, 28.4784) -> (18.4407, 27.9423) construction
  line L2311 (18.4407, 27.9423) -> (18.8752, 27.5078) construction
  line L2312 (18.8752, 27.5078) -> (19.4112, 27.5078) construction
  spline S731 degree 3 poles (19.4112, 27.5078) (19.9472, 27.5078) (20.3818, 27.9423) (20.3818, 28.4784) knots 0 0 0 0 1 1 1 1
  line L2313 (19.4112, 27.5078) -> (19.9472, 27.5078) construction
  line L2314 (19.9472, 27.5078) -> (20.3818, 27.9423) construction
  line L2315 (20.3818, 27.9423) -> (20.3818, 28.4784) construction
  spline S732 degree 3 poles (20.3818, 31.0325) (20.3818, 31.5684) (19.9472, 32.003) (19.4112, 32.003) knots 0 0 0 0 1 1 1 1
  line L2316 (20.3818, 31.0325) -> (20.3818, 31.5684) construction
  line L2317 (20.3818, 31.5684) -> (19.9472, 32.003) construction
  line L2318 (19.9472, 32.003) -> (19.4112, 32.003) construction
  spline S733 degree 3 poles (19.4112, 32.003) (18.8752, 32.003) (18.4407, 31.5684) (18.4407, 31.0325) knots 0 0 0 0 1 1 1 1
  line L2319 (19.4112, 32.003) -> (18.8752, 32.003) construction
  line L2320 (18.8752, 32.003) -> (18.4407, 31.5684) construction
  line L2321 (18.4407, 31.5684) -> (18.4407, 31.0325) construction
  spline S734 degree 3 poles (18.4407, 31.0325) (18.4407, 30.4965) (18.8752, 30.0619) (19.4112, 30.0619) knots 0 0 0 0 1 1 1 1
  line L2322 (18.4407, 31.0325) -> (18.4407, 30.4965) construction
  line L2323 (18.4407, 30.4965) -> (18.8752, 30.0619) construction
  line L2324 (18.8752, 30.0619) -> (19.4112, 30.0619) construction
  spline S735 degree 3 poles (19.4112, 30.0619) (19.9472, 30.0619) (20.3818, 30.4965) (20.3818, 31.0325) knots 0 0 0 0 1 1 1 1
  line L2325 (19.4112, 30.0619) -> (19.9472, 30.0619) construction
  line L2326 (19.9472, 30.0619) -> (20.3818, 30.4965) construction
  line L2327 (20.3818, 30.4965) -> (20.3818, 31.0325) construction
  spline S736 degree 3 poles (17.8276, 25.9242) (17.8276, 26.4602) (17.3931, 26.8948) (16.8571, 26.8948) knots 0 0 0 0 1 1 1 1
  line L2328 (17.8276, 25.9242) -> (17.8276, 26.4602) construction
  line L2329 (17.8276, 26.4602) -> (17.3931, 26.8948) construction
  line L2330 (17.3931, 26.8948) -> (16.8571, 26.8948) construction
  spline S737 degree 3 poles (16.8571, 26.8948) (16.3211, 26.8948) (15.8866, 26.4602) (15.8866, 25.9242) knots 0 0 0 0 1 1 1 1
  line L2331 (16.8571, 26.8948) -> (16.3211, 26.8948) construction
  line L2332 (16.3211, 26.8948) -> (15.8866, 26.4602) construction
  line L2333 (15.8866, 26.4602) -> (15.8866, 25.9242) construction
  spline S738 degree 3 poles (15.8866, 25.9242) (15.8866, 25.3882) (16.3211, 24.9537) (16.8571, 24.9537) knots 0 0 0 0 1 1 1 1
  line L2334 (15.8866, 25.9242) -> (15.8866, 25.3882) construction
  line L2335 (15.8866, 25.3882) -> (16.3211, 24.9537) construction
  line L2336 (16.3211, 24.9537) -> (16.8571, 24.9537) construction
  spline S739 degree 3 poles (16.8571, 24.9537) (17.3931, 24.9537) (17.8276, 25.3882) (17.8276, 25.9242) knots 0 0 0 0 1 1 1 1
  line L2337 (16.8571, 24.9537) -> (17.3931, 24.9537) construction
  line L2338 (17.3931, 24.9537) -> (17.8276, 25.3882) construction
  line L2339 (17.8276, 25.3882) -> (17.8276, 25.9242) construction
  spline S740 degree 3 poles (17.8276, 28.4784) (17.8276, 29.0143) (17.3931, 29.4489) (16.8571, 29.4489) knots 0 0 0 0 1 1 1 1
  line L2340 (17.8276, 28.4784) -> (17.8276, 29.0143) construction
  line L2341 (17.8276, 29.0143) -> (17.3931, 29.4489) construction
  line L2342 (17.3931, 29.4489) -> (16.8571, 29.4489) construction
  spline S741 degree 3 poles (16.8571, 29.4489) (16.3211, 29.4489) (15.8866, 29.0143) (15.8866, 28.4784) knots 0 0 0 0 1 1 1 1
  line L2343 (16.8571, 29.4489) -> (16.3211, 29.4489) construction
  line L2344 (16.3211, 29.4489) -> (15.8866, 29.0143) construction
  line L2345 (15.8866, 29.0143) -> (15.8866, 28.4784) construction
  spline S742 degree 3 poles (15.8866, 28.4784) (15.8866, 27.9423) (16.3211, 27.5078) (16.8571, 27.5078) knots 0 0 0 0 1 1 1 1
  line L2346 (15.8866, 28.4784) -> (15.8866, 27.9423) construction
  line L2347 (15.8866, 27.9423) -> (16.3211, 27.5078) construction
  line L2348 (16.3211, 27.5078) -> (16.8571, 27.5078) construction
  spline S743 degree 3 poles (16.8571, 27.5078) (17.3931, 27.5078) (17.8276, 27.9423) (17.8276, 28.4784) knots 0 0 0 0 1 1 1 1
  line L2349 (16.8571, 27.5078) -> (17.3931, 27.5078) construction
  line L2350 (17.3931, 27.5078) -> (17.8276, 27.9423) construction
  line L2351 (17.8276, 27.9423) -> (17.8276, 28.4784) construction
  spline S744 degree 3 poles (17.8276, 31.0325) (17.8276, 31.5684) (17.3931, 32.003) (16.8571, 32.003) knots 0 0 0 0 1 1 1 1
  line L2352 (17.8276, 31.0325) -> (17.8276, 31.5684) construction
  line L2353 (17.8276, 31.5684) -> (17.3931, 32.003) construction
  line L2354 (17.3931, 32.003) -> (16.8571, 32.003) construction
  spline S745 degree 3 poles (16.8571, 32.003) (16.3211, 32.003) (15.8866, 31.5684) (15.8866, 31.0325) knots 0 0 0 0 1 1 1 1
  line L2355 (16.8571, 32.003) -> (16.3211, 32.003) construction
  line L2356 (16.3211, 32.003) -> (15.8866, 31.5684) construction
  line L2357 (15.8866, 31.5684) -> (15.8866, 31.0325) construction
  spline S746 degree 3 poles (15.8866, 31.0325) (15.8866, 30.4965) (16.3211, 30.0619) (16.8571, 30.0619) knots 0 0 0 0 1 1 1 1
  line L2358 (15.8866, 31.0325) -> (15.8866, 30.4965) construction
  line L2359 (15.8866, 30.4965) -> (16.3211, 30.0619) construction
  line L2360 (16.3211, 30.0619) -> (16.8571, 30.0619) construction
  spline S747 degree 3 poles (16.8571, 30.0619) (17.3931, 30.0619) (17.8276, 30.4965) (17.8276, 31.0325) knots 0 0 0 0 1 1 1 1
  line L2361 (16.8571, 30.0619) -> (17.3931, 30.0619) construction
  line L2362 (17.3931, 30.0619) -> (17.8276, 30.4965) construction
  line L2363 (17.8276, 30.4965) -> (17.8276, 31.0325) construction
  spline S748 degree 3 poles (38.2606, 33.5866) (38.2606, 34.1226) (37.826, 34.5571) (37.29, 34.5571) knots 0 0 0 0 1 1 1 1
  line L2364 (38.2606, 33.5866) -> (38.2606, 34.1226) construction
  line L2365 (38.2606, 34.1226) -> (37.826, 34.5571) construction
  line L2366 (37.826, 34.5571) -> (37.29, 34.5571) construction
  spline S749 degree 3 poles (37.29, 34.5571) (36.754, 34.5571) (36.3194, 34.1226) (36.3194, 33.5866) knots 0 0 0 0 1 1 1 1
  line L2367 (37.29, 34.5571) -> (36.754, 34.5571) construction
  line L2368 (36.754, 34.5571) -> (36.3194, 34.1226) construction
  line L2369 (36.3194, 34.1226) -> (36.3194, 33.5866) construction
  spline S750 degree 3 poles (36.3194, 33.5866) (36.3194, 33.0506) (36.754, 32.616) (37.29, 32.616) knots 0 0 0 0 1 1 1 1
  line L2370 (36.3194, 33.5866) -> (36.3194, 33.0506) construction
  line L2371 (36.3194, 33.0506) -> (36.754, 32.616) construction
  line L2372 (36.754, 32.616) -> (37.29, 32.616) construction
  spline S751 degree 3 poles (37.29, 32.616) (37.826, 32.616) (38.2606, 33.0506) (38.2606, 33.5866) knots 0 0 0 0 1 1 1 1
  line L2373 (37.29, 32.616) -> (37.826, 32.616) construction
  line L2374 (37.826, 32.616) -> (38.2606, 33.0506) construction
  line L2375 (38.2606, 33.0506) -> (38.2606, 33.5866) construction
  spline S752 degree 3 poles (40.8147, 33.5866) (40.8147, 34.1226) (40.3801, 34.5571) (39.8441, 34.5571) knots 0 0 0 0 1 1 1 1
  line L2376 (40.8147, 33.5866) -> (40.8147, 34.1226) construction
  line L2377 (40.8147, 34.1226) -> (40.3801, 34.5571) construction
  line L2378 (40.3801, 34.5571) -> (39.8441, 34.5571) construction
  spline S753 degree 3 poles (39.8441, 34.5571) (39.3081, 34.5571) (38.8735, 34.1226) (38.8735, 33.5866) knots 0 0 0 0 1 1 1 1
  line L2379 (39.8441, 34.5571) -> (39.3081, 34.5571) construction
  line L2380 (39.3081, 34.5571) -> (38.8735, 34.1226) construction
  line L2381 (38.8735, 34.1226) -> (38.8735, 33.5866) construction
  spline S754 degree 3 poles (38.8735, 33.5866) (38.8735, 33.0506) (39.3081, 32.616) (39.8441, 32.616) knots 0 0 0 0 1 1 1 1
  line L2382 (38.8735, 33.5866) -> (38.8735, 33.0506) construction
  line L2383 (38.8735, 33.0506) -> (39.3081, 32.616) construction
  line L2384 (39.3081, 32.616) -> (39.8441, 32.616) construction
  spline S755 degree 3 poles (39.8441, 32.616) (40.3801, 32.616) (40.8147, 33.0506) (40.8147, 33.5866) knots 0 0 0 0 1 1 1 1
  line L2385 (39.8441, 32.616) -> (40.3801, 32.616) construction
  line L2386 (40.3801, 32.616) -> (40.8147, 33.0506) construction
  line L2387 (40.8147, 33.0506) -> (40.8147, 33.5866) construction
  spline S756 degree 3 poles (43.3688, 33.5866) (43.3688, 34.1226) (42.9342, 34.5571) (42.3982, 34.5571) knots 0 0 0 0 1 1 1 1
  line L2388 (43.3688, 33.5866) -> (43.3688, 34.1226) construction
  line L2389 (43.3688, 34.1226) -> (42.9342, 34.5571) construction
  line L2390 (42.9342, 34.5571) -> (42.3982, 34.5571) construction
  spline S757 degree 3 poles (42.3982, 34.5571) (41.8622, 34.5571) (41.4277, 34.1226) (41.4277, 33.5866) knots 0 0 0 0 1 1 1 1
  line L2391 (42.3982, 34.5571) -> (41.8622, 34.5571) construction
  line L2392 (41.8622, 34.5571) -> (41.4277, 34.1226) construction
  line L2393 (41.4277, 34.1226) -> (41.4277, 33.5866) construction